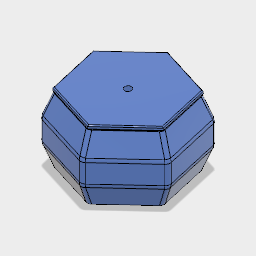
Mikan v2 (Autodesk Fusion 360 design; units mm, degrees)
Autodesk Fusion 360 part; units mm, degrees
sketch "Sketch1" plane through (0, 0, 0) normal (0, 1, 0) x (1, 0, 0)
  line L0 (50.7455, -15.6915) -> (38.962, 36.1012)
  line L1 (38.962, 36.1012) -> (-11.7835, 51.7927)
  line L2 (-11.7835, 51.7927) -> (-50.7455, 15.6915)
  line L3 (-50.7455, 15.6915) -> (-38.962, -36.1012)
  line L4 (-38.962, -36.1012) -> (11.7835, -51.7927)
  line L5 (11.7835, -51.7927) -> (50.7455, -15.6915)
  dimension "d1" = 46
  measures "d1" distance of origin L5
extrude "Extrude1" add sketch "Sketch1" along normal blind 21 draft 20 makes body 1
ref_plane "WorkPlane1" through (0, 21, 0) normal (0, 1, 0) x (1, 0, 0)
mirror "Mirror1" about plane through (0, 21, 0) normal (0, 1, 0) of bodies 1 makes body 2
move_body "Move1" bodies 2 to x (1, 0, 0) y (0, 1, 0) z (0, 0, 1) at (0, 80, 0)
sketch "Sketch2" plane through (0, 21, 0) normal (0, 1, 0) x (1, 0, 0)
extrude "Extrude2" add 1 faces at (-15.1453, 21, 14.0333) along direction (0, 1, 0) blind 22 on bodies 1 bodies 1
move_body "Move2" bodies 2 to x (1, 0, 0) y (0, 1, 0) z (0, 0, 1) at (0, -58, 0)
combine "Combine1" operation add target body 2 tool bodies 1
ref_plane "WorkPlane2" through (0, 64, 0) normal (0, 1, 0) x (-1, 0, 0)
sketch "Sketch3" plane through (0, 64, 0) normal (0, 1, 0) x (1, 0, 0)
  line L0 (-11.7835, 51.7927) -> (-50.7455, 15.6915)
  line L1 (-11.7835, 51.7927) -> (-50.7455, 15.6915)
  line L2 (-38.962, -36.1012) -> (11.7835, -51.7927)
  line L3 (-38.962, -36.1012) -> (11.7835, -51.7927)
  line L4 (50.7455, -15.6915) -> (11.7835, -51.7927)
  line L5 (-50.7455, 15.6915) -> (-38.962, -36.1012)
  line L6 (-38.962, -36.1012) -> (-50.7455, 15.6915)
  line L7 (38.962, 36.1012) -> (-11.7835, 51.7927)
  line L8 (-11.7835, 51.7927) -> (38.962, 36.1012)
  line L9 (50.7455, -15.6915) -> (38.962, 36.1012)
  line L10 (50.7455, -15.6915) -> (38.962, 36.1012)
  line L11 (33.0827, -32.0575) -> (31.0437, -29.8569)
  line L12 (43.8382, 14.6687) -> (40.9129, 14.0032)
  line L13 (16.5085, 43.0442) -> (15.6222, 40.1781)
  line L14 (-29.5282, 35.3509) -> (-27.4892, 33.1503)
  line L15 (-44.8538, -10.2048) -> (-41.9285, -9.5393)
  line L16 (-13.5892, -43.9469) -> (-12.703, -41.0808)
  line L17 (31.0437, -29.8569) -> (13.2963, -46.3012)
  line L18 (-12.703, -41.0808) -> (13.0177, -49.0342)
  line L19 (13.2963, -46.3012) -> (11.015, -48.4149)
  line L20 (31.0437, -29.8569) -> (48.6799, -13.5156)
  line L21 (40.9129, 14.0032) -> (47.436, -14.6682)
  line L22 (40.9129, 14.0032) -> (35.8469, 36.2702)
  line L23 (15.6222, 40.1781) -> (36.421, 33.7467)
  line L24 (15.6222, 40.1781) -> (-12.2714, 48.8034)
  line L25 (-27.4892, 33.1503) -> (-11.015, 48.4149)
  line L26 (-27.4892, 33.1503) -> (-49.1997, 13.034)
  line L27 (-41.9285, -9.5393) -> (-47.436, 14.6682)
  line L28 (-41.9285, -9.5393) -> (-36.0292, -35.4688)
  line L29 (-12.703, -41.0808) -> (-36.421, -33.7467)
  point P0 (-11.7835, 51.7927)
  point P1 (-50.7455, 15.6915)
  point P2 (-38.962, -36.1012)
  point P3 (11.7835, -51.7927)
  point P4 (50.7455, -15.6915)
  point P5 (11.7835, -51.7927)
  point P6 (-38.962, -36.1012)
  point P7 (-50.7455, 15.6915)
  point P8 (-11.7835, 51.7927)
  point P9 (38.962, 36.1012)
  point P10 (38.962, 36.1012)
  dimension "d15" = 3
  dimension "d16" = 3
  dimension "d17" = 3
  dimension "d18" = 3
  dimension "d20" = 3
  dimension "d21" = 3
  measures "d15" distance of L11.start L11.end
  measures "d16" distance of L12.start L12.end
  measures "d17" distance of L13.start L13.end
  measures "d18" distance of L14.start L14.end
  measures "d20" distance of L15.start L15.end
  measures "d21" distance of L16.start L16.end
extrude "Extrude3" cut sketch "Sketch3" against normal blind 60 contours L17 L18 L19 L20 L21 L22 L23 L24 L25 L26 L27 L28 L29 bodies 2
fillet "Fillet1" radius 10 1 edges at (52.3067, 43, -11.9005) on bodies 2
fillet "Fillet2" radius 10 11 edges at (52.3067, 21, -11.9005) (15.8472, 21, -51.2492) (15.7608, 43, -51.2759) (36.3931, 43, 39.4102) (36.4595, 21, 39.3487) (-36.4595, 43, -39.3487) (-52.3067, 43, 11.9005) (-52.3067, 21, 11.9005) (-36.4595, 21, -39.3487) (-15.8472, 43, 51.2492) (-15.8472, 21, 51.2492) on bodies 2
fillet "Fillet3" radius 5 30 edges at (54.6288, 54.3285, 16.8923) (59.0098, 42.9732, 18.247) (59.1774, 32, 18.2988) (59.0098, 21.0268, 18.247) (54.6288, 9.6715, 16.8923) (-41.9436, 9.6715, 38.8638) (-45.3073, 21.0268, 41.9805) (-45.436, 32, 42.0998) (-45.3073, 42.9732, 41.9805) (-41.9436, 54.3285, 38.8638) (12.6853, 54.3285, 55.7561) (13.7026, 42.9732, 60.2275) (13.7415, 32, 60.3986) (13.7026, 21.0268, 60.2275) (12.6853, 9.6715, 55.7561) (-54.6288, 54.3285, -16.8923) (-59.0098, 42.9732, -18.247) (-59.1774, 32, -18.2988) (-59.0098, 21.0268, -18.247) (-54.6288, 9.6715, -16.8923) (41.9436, 54.3285, -38.8638) (45.3073, 42.9732, -41.9805) (45.436, 32, -42.0998) (45.3073, 21.0268, -41.9805) (41.9436, 9.6715, -38.8638) (-12.6853, 54.3285, -55.7561) (-13.7026, 42.9732, -60.2275) (-13.7415, 32, -60.3986) (-13.7026, 21.0268, -60.2275) (-12.6853, 9.6715, -55.7561) on bodies 2
ref_plane "WorkPlane3" through (0, 61, 0) normal (0, 1, 0) x (-1, 0, 0)
sketch "Sketch4" plane through (0, 61, 0) normal (0, 1, 0) x (1, 0, 0)
  line L0 (36.3704, 36.9025) -> (-9.1919, 50.9913)
  line L1 (-11.015, 48.4149) -> (36.421, 33.7467)
  line L2 (36.421, 33.7467) -> (47.436, -14.6682)
  line L3 (36.421, 33.7467) -> (47.436, -14.6682)
  line L4 (11.015, -48.4149) -> (47.436, -14.6682)
  line L5 (11.015, -48.4149) -> (-36.421, -33.7467)
  line L6 (11.015, -48.4149) -> (-36.421, -33.7467)
  line L7 (-36.421, -33.7467) -> (-47.436, 14.6682)
  line L8 (-47.436, 14.6682) -> (-11.015, 48.4149)
  point P0 (-11.015, 48.4149)
  point P1 (36.421, 33.7467)
  point P2 (47.436, -14.6682)
  point P3 (11.015, -48.4149)
  point P4 (11.015, -48.4149)
  point P5 (-36.421, -33.7467)
  point P6 (-47.436, 14.6682)
extrude "Extrude4" add sketch "Sketch4" along normal blind 3 separate body makes body 3
ref_plane "WorkPlane4" through (0, 64, 0) normal (0, 1, 0) x (0, 0, 1)
sketch "Sketch5" plane through (0, 64, 0) normal (0, 1, 0) x (1, 0, 0)
  line L0 (-38.962, -36.1012) -> (11.7835, -51.7927)
  line L1 (11.7835, -51.7927) -> (50.7455, -15.6915)
  line L2 (50.7455, -15.6915) -> (38.962, 36.1012)
  line L3 (38.962, 36.1012) -> (-11.7835, 51.7927)
  line L4 (-11.7835, 51.7927) -> (-50.7455, 15.6915)
  line L5 (-50.7455, 15.6915) -> (-38.962, -36.1012)
extrude "Extrude5" add sketch "Sketch5" along normal blind 4 bodies 3
fillet "Fillet4" radius 1 12 edges at (-31.2645, 68, -33.7421) (13.5892, 68, -43.9469) (44.8538, 68, -10.2048) (31.2645, 68, 33.7421) (31.2645, 64, 33.7421) (44.8538, 64, -10.2048) (-13.5892, 64, 43.9469) (-44.8538, 64, 10.2048) (-44.8538, 68, 10.2048) (-13.5892, 68, 43.9469) (13.5892, 64, -43.9469) (-31.2645, 64, -33.7421) on bodies 3
ref_plane "WorkPlane5" through (0, 68, 0) normal (0, 1, 0) x (0, 0, 1)
sketch "Sketch6" plane through (0, 68, 0) normal (0, 1, 0) x (1, 0, 0)
  circle A0 centre (0, 0) radius 3.5
  dimension "d35" = 7
  measures "d35" diameter of A0
extrude "Extrude6" cut sketch "Sketch6" against normal up to surface (7 mm away) bodies 3
